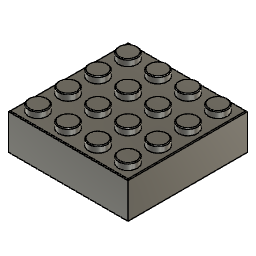
4x4block (Autodesk Fusion 360 design; units mm, degrees)
Autodesk Fusion 360 part; units mm, degrees
sketch "Sketch1" plane through (0, 0, 0) normal (0, 0, 1) x (1, 0, 0)
  line L0 (0, 0) -> (31.8, 0)
  line L1 (31.8, 0) -> (31.8, 31.8)
  line L2 (31.8, 31.8) -> (0, 31.8)
  line L3 (0, 31.8) -> (0, 0)
  constraint coincident L0.start L3.end
extrude "Extrude1" add sketch "Sketch1" along normal blind 9.6
sketch "Sketch2" plane through (0, 0, 9.6) normal (0, 0, 1) x (-1, 0, 0)
  line L0 (0, -31.8) -> (0, 0)
  line L1 (0, 0) -> (-31.8, 0)
  line L2 (-31.8, 0) -> (-31.8, -31.8)
  line L3 (-31.8, -31.8) -> (0, -31.8)
  circle A0 centre (-3.9, -27.9) radius 2.5
extrude "Extrude2" add sketch "Sketch2" along normal blind 1.7 contours A0
pattern_linear "R-Pattern1" count 4 spacing 8 along (1, 0, 0) count 4 spacing 8 along (0, -1, 0) of "Extrude2"
shell "Shell1" thickness 1.49 removed faces 1 at (10.6, 21.2, 0)
sketch "Sketch3" plane through (0, 0, 8.11) normal (0, 0, -1) x (1, 0, 0)
  circle A0 centre (27.9, -3.9) radius 1.01
  circle A1 centre (19.9, -3.9) radius 1.01
  circle A2 centre (11.9, -3.9) radius 1.01
  circle A3 centre (3.9, -3.9) radius 1.01
  circle A4 centre (27.9, -11.9) radius 1.01
  circle A5 centre (19.9, -11.9) radius 1.01
  circle A6 centre (11.9, -11.9) radius 1.01
  circle A7 centre (3.9, -11.9) radius 1.01
  circle A8 centre (27.9, -19.9) radius 1.01
  circle A9 centre (19.9, -19.9) radius 1.01
  circle A10 centre (11.9, -19.9) radius 1.01
  circle A11 centre (3.9, -19.9) radius 1.01
  circle A12 centre (27.9, -27.9) radius 1.01
  circle A13 centre (19.9, -27.9) radius 1.01
  circle A14 centre (11.9, -27.9) radius 1.01
  circle A15 centre (3.9, -27.9) radius 1.01
  line L0 (1.49, -1.49) -> (1.49, -30.31)
  line L1 (1.49, -30.31) -> (30.31, -30.31)
  line L2 (30.31, -30.31) -> (30.31, -1.49)
  line L3 (30.31, -1.49) -> (1.49, -1.49)
  circle A16 centre (7.9, -7.9) radius 3.15
  circle A17 centre (7.9, -7.9) radius 2.15
extrude "Extrude3" add sketch "Sketch3" along normal blind 8.1 contours A16
pattern_linear "R-Pattern2" count 3 spacing 8 along (1, 0, 0) count 3 spacing 8 along (0, 1, 0) of "Extrude3"
fillet "Fillet1" radius 0.2 20 edges at (0, 15.9, 9.6) (15.9, 31.8, 9.6) (31.8, 15.9, 9.6) (15.9, 0, 9.6) (30.2308, 4.804, 11.3) (22.2308, 4.804, 11.3) (14.2308, 4.804, 11.3) (6.2308, 4.804, 11.3) (6.2308, 12.804, 11.3) (14.2308, 12.804, 11.3) (22.2308, 12.804, 11.3) (30.2308, 12.804, 11.3) (30.2308, 20.804, 11.3) (22.2308, 20.804, 11.3) (14.2308, 20.804, 11.3) (6.2308, 20.804, 11.3) (6.2308, 28.804, 11.3) (14.2308, 28.804, 11.3) (22.2308, 28.804, 11.3) (30.2308, 28.804, 11.3)
scale "Scale1" factor 0.75 about (30.2, 27.9, 11.3) bodies 1
